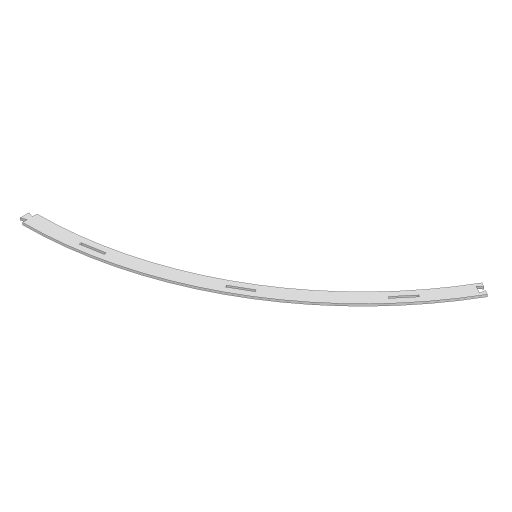
# Autodesk Inventor part: D90_CM_CIRCULO
Saved by Autodesk Inventor 2024.2 (Build 282272000, 272)
## iProperties
Created: 2024-10-01
Part Number: D90_CM_CIRCULO
Material: Generic
Document SubType Name: Modeling
Designer: jrcer
Density: 1 g/cm^3
Appearance: Default
Author: jrcer
Autodesk Inventor part; units mm, degrees
ref_plane "YZ Plane" through (0, 0, 0) normal (1, 0, 0) x (0, 1, 0)
ref_plane "XZ Plane" through (0, 0, 0) normal (0, 1, 0) x (-1, 0, 0)
ref_plane "XY Plane" through (0, 0, 0) normal (0, 0, 1) x (1, 0, 0)
sketch "Sketch1" plane through (0, 0, 0) normal (0, 1, 0) x (-1, 0, 0)
  circle A0 centre (0, 0) radius 450
  circle A1 centre (0, 0) radius 470
  line L0 (470, 0) -> (450, 0)
  line L1 (-470, 0) -> (-450, 0)
  line L2 (0, 0) -> (-389.7114, 225) construction
  line L3 (0, 450) -> (0, 0) construction
  line L4 (0, 470) -> (0, 450)
  line L5 (-389.7114, 225) -> (-407.0319, 235)
  line L6 (-389.6755, 233.0622) -> (-400.0678, 239.0622)
  line L7 (-400.0678, 239.0622) -> (-401.3614, 231.7261)
  line L8 (-389.6755, 233.0622) -> (-395.382, 228.2739)
  line L9 (-398.3717, 230) -> (-394.8717, 236.0622) construction
  line L10 (7, 454) -> (0, 456.5478)
  line L11 (7, 454) -> (7, 466)
  line L12 (7, 466) -> (0, 463.4522)
  line L13 (396.6755, 220.9378) -> (395.382, 228.2739)
  line L14 (396.6755, 220.9378) -> (407.0678, 226.9378)
  line L15 (407.0678, 226.9378) -> (401.3614, 231.7261)
  line L16 (389.6755, -233.0622) -> (395.382, -228.2739)
  line L17 (389.6755, -233.0622) -> (400.0678, -239.0622)
  line L18 (400.0678, -239.0622) -> (401.3614, -231.7261)
  line L19 (-7, -454) -> (0, -456.5478)
  line L20 (-7, -454) -> (-7, -466)
  line L21 (-7, -466) -> (0, -463.4522)
  line L22 (-396.6755, -220.9378) -> (-395.382, -228.2739)
  line L23 (-396.6755, -220.9378) -> (-407.0678, -226.9378)
  line L24 (-407.0678, -226.9378) -> (-401.3614, -231.7261)
  line L25 (-363.084, 285.1192) -> (-343.7989, 308.0994)
  line L26 (-343.7989, 308.0994) -> (-341.3477, 306.0423)
  line L27 (-341.3477, 306.0423) -> (-360.6327, 283.0622)
  line L28 (-360.6327, 283.0622) -> (-363.084, 285.1192)
  line L29 (-363.084, 285.1192) -> (-341.3477, 306.0423) construction
  line L30 (-343.7989, 308.0994) -> (-360.6327, 283.0622) construction
  circle A2 centre (0, 0) radius 460.0533 construction
  line L31 (-435.6969, 142.6478) -> (-438.7038, 143.7424)
  line L32 (-438.7038, 143.7424) -> (-428.4415, 171.9326)
  line L33 (-425.4346, 170.8379) -> (-435.6969, 142.6478)
  line L34 (-428.4415, 171.9326) -> (-425.4346, 170.8379)
  line L35 (-458.2096, -14.9721) -> (-461.4096, -14.9719)
  line L36 (-461.4096, -14.9719) -> (-461.4077, 15.0281)
  line L37 (-458.2077, 15.0279) -> (-458.2096, -14.9721)
  line L38 (-461.4077, 15.0281) -> (-458.2077, 15.0279)
  line L39 (-425.4554, -170.786) -> (-428.4625, -171.8803)
  line L40 (-428.4625, -171.8803) -> (-438.7214, -143.6889)
  line L41 (-435.7143, -142.5946) -> (-425.4554, -170.786)
  line L42 (-438.7214, -143.6889) -> (-435.7143, -142.5946)
  line L43 (-341.385, -306.0007) -> (-343.8365, -308.0575)
  line L44 (-343.8365, -308.0575) -> (-363.1187, -285.075)
  line L45 (-360.6673, -283.0182) -> (-341.385, -306.0007)
  line L46 (-363.1187, -285.075) -> (-360.6673, -283.0182)
  line L47 (-216.1386, -404.3072) -> (-217.7388, -407.0783)
  line L48 (-217.7388, -407.0783) -> (-243.7186, -392.0768)
  line L49 (-242.1185, -389.3056) -> (-216.1386, -404.3072)
  line L50 (-243.7186, -392.0768) -> (-242.1185, -389.3056)
  line L51 (-64.8227, -453.8482) -> (-65.3785, -456.9996)
  line L52 (-65.3785, -456.9996) -> (-94.9224, -451.7883)
  line L53 (-94.3666, -448.637) -> (-64.8227, -453.8482)
  line L54 (-94.9224, -451.7883) -> (-94.3666, -448.637)
  line L55 (94.3118, -448.6485) -> (94.8673, -451.7999)
  line L56 (94.8673, -451.7999) -> (65.3228, -457.0075)
  line L57 (64.7673, -453.8561) -> (94.3118, -448.6485)
  line L58 (65.3228, -457.0075) -> (64.7673, -453.8561)
  line L59 (242.071, -389.3351) -> (243.6708, -392.1065)
  line L60 (243.6708, -392.1065) -> (217.6891, -407.1049)
  line L61 (216.0893, -404.3335) -> (242.071, -389.3351)
  line L62 (217.6891, -407.1049) -> (216.0893, -404.3335)
  line L63 (360.6327, -283.0622) -> (363.084, -285.1192)
  line L64 (363.084, -285.1192) -> (343.7989, -308.0994)
  line L65 (341.3477, -306.0423) -> (360.6327, -283.0622)
  line L66 (343.7989, -308.0994) -> (341.3477, -306.0423)
  line L67 (435.6969, -142.6478) -> (438.7038, -143.7424)
  line L68 (438.7038, -143.7424) -> (428.4415, -171.9326)
  line L69 (425.4346, -170.8379) -> (435.6969, -142.6478)
  line L70 (428.4415, -171.9326) -> (425.4346, -170.8379)
  line L71 (458.2096, 14.9721) -> (461.4096, 14.9719)
  line L72 (461.4096, 14.9719) -> (461.4077, -15.0281)
  line L73 (458.2077, -15.0279) -> (458.2096, 14.9721)
  line L74 (461.4077, -15.0281) -> (458.2077, -15.0279)
  line L75 (425.4554, 170.786) -> (428.4625, 171.8803)
  line L76 (428.4625, 171.8803) -> (438.7214, 143.6889)
  line L77 (435.7143, 142.5946) -> (425.4554, 170.786)
  line L78 (438.7214, 143.6889) -> (435.7143, 142.5946)
  line L79 (341.385, 306.0007) -> (343.8365, 308.0575)
  line L80 (343.8365, 308.0575) -> (363.1187, 285.075)
  line L81 (360.6673, 283.0182) -> (341.385, 306.0007)
  line L82 (363.1187, 285.075) -> (360.6673, 283.0182)
  line L83 (216.1386, 404.3072) -> (217.7388, 407.0783)
  line L84 (217.7388, 407.0783) -> (243.7186, 392.0768)
  line L85 (242.1185, 389.3056) -> (216.1386, 404.3072)
  line L86 (243.7186, 392.0768) -> (242.1185, 389.3056)
  line L87 (64.8227, 453.8482) -> (65.3785, 456.9996)
  line L88 (65.3785, 456.9996) -> (94.9224, 451.7883)
  line L89 (94.3666, 448.637) -> (64.8227, 453.8482)
  line L90 (94.9224, 451.7883) -> (94.3666, 448.637)
  line L91 (-94.3118, 448.6485) -> (-94.8673, 451.7999)
  line L92 (-94.8673, 451.7999) -> (-65.3228, 457.0075)
  line L93 (-64.7673, 453.8561) -> (-94.3118, 448.6485)
  line L94 (-65.3228, 457.0075) -> (-64.7673, 453.8561)
  line L95 (-242.071, 389.3351) -> (-243.6708, 392.1065)
  line L96 (-243.6708, 392.1065) -> (-217.6891, 407.1049)
  line L97 (-216.0893, 404.3335) -> (-242.071, 389.3351)
  line L98 (-217.6891, 407.1049) -> (-216.0893, 404.3335)
  point P0 (460, 0)
  point P1 (-460, 0)
  point P2 (7, 460)
  point P3 (401.8717, 223.9378)
  point P4 (394.8717, -236.0622)
  point P5 (-7, -460)
  point P6 (-401.8717, -223.9378)
  point P7 (-352.2158, 295.5808)
  point P8 (7, 460)
  point P9 (-361.8584, 284.0907)
  point P10 (-342.5733, 307.0709)
  point P11 (-437.2004, 143.1951)
  point P12 (-426.938, 171.3853)
  point P13 (-459.8096, -14.972)
  point P14 (-459.8077, 15.028)
  point P15 (-426.959, -171.3332)
  point P16 (-437.2178, -143.1418)
  point P17 (-342.6108, -307.0291)
  point P18 (-361.893, -284.0466)
  point P19 (-216.9387, -405.6927)
  point P20 (-242.9185, -390.6912)
  point P21 (-65.1006, -455.4239)
  point P22 (-94.6445, -450.2126)
  point P23 (94.5896, -450.2242)
  point P24 (65.045, -455.4318)
  point P25 (242.8709, -390.7208)
  point P26 (216.8892, -405.7192)
  point P27 (361.8584, -284.0907)
  point P28 (342.5733, -307.0709)
  point P29 (437.2004, -143.1951)
  point P30 (426.938, -171.3853)
  point P31 (459.8096, 14.972)
  point P32 (459.8077, -15.028)
  point P33 (426.959, 171.3332)
  point P34 (437.2178, 143.1418)
  point P35 (342.6108, 307.0291)
  point P36 (361.893, 284.0466)
  point P37 (216.9387, 405.6927)
  point P38 (242.9185, 390.6912)
  point P39 (65.1006, 455.4239)
  point P40 (94.6445, 450.2126)
  point P41 (-94.5896, 450.2242)
  point P42 (-65.045, 455.4318)
  point P43 (-242.8709, 390.7208)
  point P44 (-216.8892, 405.7192)
  dimension "d0" = 900
  dimension "d1" = 940
  dimension "d4" = 60
  dimension "d5" = 7
  dimension "d6" = 70
  dimension "d8" = 12
  dimension "d11" = 360
  dimension "d13" = 3.2
  dimension "d14" = 30
  dimension "d15" = 50
  dimension "d18" = 360
  constraints: 198 end point, 11 point on circle, 9 midpoint, 3 centre point, 3 coincident, 3 parallel, 2 horizontal, 2 horizontal alignment, 2 perpendicular, 2 point on line, 2 vertical, 1 collinear, 1 equal length, 230 other
  measures "d0" diameter of A0
  measures "d1" diameter of A1
  measures "d4" angle of L2 L3
  measures "d5" distance between parallel lines of L6 L5
  measures "d6" angle of L7 L6
  measures "d8" distance of L6.start L6.end
  measures "d13" distance of L25.end L26.end
  measures "d14" distance of L26.end L27.end
  measures "d15" vertical distance of L27.end L6.start
extrude "Extrusion1" add sketch "Sketch1" along normal blind 3 contours A0 L5 L8 L6 L7 A1 L4 | L4 L12 L11 L10
body "Solid1"
